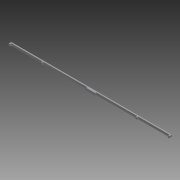
# Autodesk Inventor part: connection
Saved by Autodesk Inventor 2011 (Build 150239000, 239)
## iProperties
Created: 2011-07-10
Part Number: connection
Document SubType Name: Modeling
Designer: adowning
Density: 1 g/cm^3
Author: adowning
Autodesk Inventor part; units mm, degrees
ref_plane "YZ Plane" through (0, 0, 0) normal (1, 0, 0) x (0, 1, 0)
ref_plane "XZ Plane" through (0, 0, 0) normal (0, 1, 0) x (-1, 0, 0)
ref_plane "XY Plane" through (0, 0, 0) normal (0, 0, 1) x (1, 0, 0)
sketch "Sketch1" plane through (0, 0, 0) normal (0, 0, 1) x (1, 0, 0)
  line L0 (-44.3649, 2.907) -> (399.3477, 2.907)
  line L1 (399.3477, 2.907) -> (399.3477, -3.443)
  line L2 (399.3477, -3.443) -> (-44.3649, -3.443)
  line L3 (-44.3649, -3.443) -> (-44.3649, 2.907)
  point P0 (0, 0)
  dimension "d0" = 443.7126
  dimension "d1" = 6.35
  constraints: 8 end point, 2 parallel, 1 horizontal, 1 perpendicular
  measures "d0" distance of L1.end L2.end
  measures "d1" distance of L0.end L1.end
extrude "Extrusion1" add sketch "Sketch1" along normal blind 3.175
sketch "Sketch2" plane through (0, 0, 3.175) normal (0, 0, 1) x (1, 0, 0)
  line L0 (399.3477, 2.907) -> (399.3477, -3.443) projected
  line L1 (-44.3649, 2.907) -> (399.3477, 2.907) projected
  line L2 (-44.3649, -3.443) -> (-44.3649, 2.907) projected
  line L3 (-44.3649, 2.907) -> (-44.3649, -0.268)
  line L4 (-44.3649, -0.268) -> (399.3477, -0.268)
  line L5 (399.3477, -0.268) -> (309.6603, -0.268)
  line L6 (-44.3649, -0.268) -> (45.3225, -0.268)
  circle A0 centre (-44.3649, -0.268) radius 3.175
  circle A1 centre (45.3225, -0.268) radius 3.175
  circle A2 centre (309.6603, -0.268) radius 3.175
  circle A3 centre (399.3477, -0.268) radius 3.175
  point P0 (0, 0)
  dimension "d4" = 3.175
  dimension "d5" = 89.6874
  dimension "d6" = 89.6874
  constraints: 8 end point, 4 coincident, 2 centre point, 2 midpoint, 2 point on line, 2 tangent, 2 vertical alignment, 4 other
  measures "d4" distance of L1.start L3.end
  measures "d5" distance of L4.end L5.end
  measures "d6" distance of L3.end L6.end
extrude "Extrusion2" add sketch "Sketch2" along normal blind 3.175 contours A3 L0 | L0 L4 A3 | L0 A3 L4 | A2 L4 | A1 L4 | A2 L4 | A0 L4 L2 | L2 A0 | A1 L4 | L4 A0 L2
sketch "Sketch3" plane through (0, 0, 3.175) normal (0, 0, -1) x (-1, 0, 0)
  line L0 (-399.3477, 2.907) -> (-399.3477, -3.443) projected
  arc A0 (-399.3477, 2.907) -> (-399.3477, -3.443) centre (-399.3477, -0.268) ccw projected
  point P0 (0, 0)
extrude "Extrusion3" add sketch "Sketch3" along normal blind 3.175
sketch "Sketch4" plane through (0, 0, 3.175) normal (0, 0, -1) x (-1, 0, 0)
  line L0 (44.3649, -3.443) -> (44.3649, 2.907) projected
  arc A0 (44.3649, -3.443) -> (44.3649, 2.907) centre (44.3649, -0.268) ccw projected
  point P0 (0, 0)
extrude "Extrusion4" add sketch "Sketch4" along normal blind 3.175
sketch "Sketch5" plane through (0, 0, 3.175) normal (0, 0, 1) x (1, 0, 0)
  arc A0 (45.3225, -3.443) -> (45.3225, 2.907) centre (45.3225, -0.268) ccw projected
  line L0 (309.6603, -3.443) -> (45.3225, -3.443) projected
  arc A1 (309.6603, 2.907) -> (309.6603, -3.443) centre (309.6603, -0.268) ccw projected
  line L1 (45.3225, 2.907) -> (309.6603, 2.907) projected
  line L2 (309.6603, -3.443) -> (45.3225, 2.907)
  line L3 (45.3225, -3.443) -> (309.6603, 2.907)
  line L4 (177.4914, -0.268) -> (177.4914, -3.443)
  line L5 (181.9749, -3.443) -> (194.6749, -3.443)
  line L6 (194.6749, -3.443) -> (169.2749, -3.443)
  line L7 (169.2749, -3.443) -> (169.2749, 2.907)
  line L8 (169.2749, 2.907) -> (194.6749, 2.907)
  line L9 (194.6749, 2.907) -> (194.6749, -3.443)
  point P0 (0, 0)
  dimension "d13" = 12.7
  dimension "d14" = 25.4
  constraints: 16 end point, 3 point on line, 2 midpoint, 2 parallel, 1 horizontal, 1 perpendicular, 2 other
  measures "d13" distance of L5.start L5.end
  measures "d14" distance of L7.end L8.end
extrude "Extrusion5" add sketch "Sketch5" along normal blind 3.175 contours L7 L3 L4 L0 | L7 L2 L3 | L1 L9 L3 L2 L7 | L4 L2 L9 L0 | L3 L9 L2
body "Solid1"
